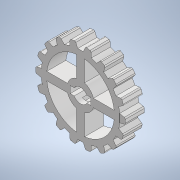
# Autodesk Inventor part: mixer_gear
Saved by Autodesk Inventor 2022 (Build 260153000, 153)
## iProperties
Created: 2022-06-21
Part Number: mixer_gear
Material: Generic
Document SubType Name: Modeling
Designer: efred
Density: 1 g/cm^3
Appearance: Default
Author: efred
Autodesk Inventor part; units mm, degrees
ref_plane "YZ Plane" through (0, 0, 0) normal (1, 0, 0) x (0, 1, 0)
ref_plane "XZ Plane" through (0, 0, 0) normal (0, 1, 0) x (-1, 0, 0)
sketch "Sketch1" plane through (0, 0, 0) normal (0, 0, 1) x (1, 0, 0)
  circle A0 centre (0, 0) radius 0.5 projected
  line L0 (-1.1547, -2) -> (-1.7321, -1) projected
  line L1 (-1.7321, -1) -> (-3.5, -1) projected
  line L2 (-3.5, -1) -> (-3.5, 1) projected
  line L3 (-3.5, 1) -> (-1.7321, 1) projected
  line L4 (-1.7321, 1) -> (-1.1547, 2) projected
  line L5 (-1.1547, 2) -> (1.1547, 2) projected
  line L6 (1.1547, 2) -> (1.7321, 1) projected
  line L7 (1.7321, 1) -> (3.5, 1) projected
  line L8 (3.5, 1) -> (3.5, -1) projected
  line L9 (3.5, -1) -> (1.7321, -1) projected
  line L10 (1.7321, -1) -> (1.1547, -2) projected
  line L11 (1.1547, -2) -> (-1.1547, -2) projected
  circle A1 centre (0, 0) radius 5
  line L12 (-3.8, -1.3) -> (-1.9053, -1.3)
  line L13 (-1.9053, -1.3) -> (-1.3279, -2.3)
  line L14 (-1.3279, -2.3) -> (1.3279, -2.3)
  line L15 (1.3279, -2.3) -> (1.9053, -1.3)
  line L16 (1.9053, -1.3) -> (3.8, -1.3)
  line L17 (3.8, -1.3) -> (3.8, 1.3)
  line L18 (3.8, 1.3) -> (1.9053, 1.3)
  line L19 (1.9053, 1.3) -> (1.3279, 2.3)
  line L20 (1.3279, 2.3) -> (-1.3279, 2.3)
  line L21 (-1.3279, 2.3) -> (-1.9053, 1.3)
  line L22 (-1.9053, 1.3) -> (-3.8, 1.3)
  line L23 (-3.8, 1.3) -> (-3.8, -1.3)
  dimension "d0" = 10
  dimension "d1" = 0.3
  constraints: 24 end point, 1 centre point, 1 coincident, 11 other
  measures "d0" diameter of A1
  measures "d1" distance between parallel lines of L1 L12
extrude "Extrusion1" add sketch "Sketch1" along normal blind 2 and the other way blind 5 contours A1
sketch "Sketch2" plane through (0, 0, -5) normal (0, 0, -1) x (-1, 0, 0)
  circle A0 centre (0, 0) radius 5 projected
  line L0 (3.8, 1.3) -> (3.8, -1.3) projected
  line L1 (3.8, -1.3) -> (1.9053, -1.3) projected
  line L2 (1.9053, -1.3) -> (1.3279, -2.3) projected
  line L3 (1.3279, -2.3) -> (-1.3279, -2.3) projected
  line L4 (-1.3279, -2.3) -> (-1.9053, -1.3) projected
  line L5 (-1.9053, -1.3) -> (-3.8, -1.3) projected
  line L6 (-3.8, -1.3) -> (-3.8, 1.3) projected
  line L7 (-3.8, 1.3) -> (-1.9053, 1.3) projected
  line L8 (-1.9053, 1.3) -> (-1.3279, 2.3) projected
  line L9 (-1.3279, 2.3) -> (1.3279, 2.3) projected
  line L10 (1.3279, 2.3) -> (1.9053, 1.3) projected
  line L11 (1.9053, 1.3) -> (3.8, 1.3) projected
  line L12 (3.8, 1.3) -> (3.8, -1.3) projected
  line L13 (3.8, 1.3) -> (3.8, -1.3)
  line L14 (3.8, -1.3) -> (1.9053, -1.3)
  line L15 (1.9053, -1.3) -> (1.3279, -2.3) projected
  line L16 (1.9053, -1.3) -> (1.3279, -2.3)
  line L17 (-1.9053, -1.3) -> (-1.3279, -2.3) projected
  line L18 (-1.3279, -2.3) -> (1.3279, -2.3)
  line L19 (1.9053, 1.3) -> (3.8, 1.3) projected
  line L20 (3.8, 1.3) -> (1.9053, 1.3)
  line L21 (1.3279, 2.3) -> (1.9053, 1.3) projected
  line L22 (1.9053, 1.3) -> (1.3279, 2.3)
  line L23 (1.3279, 2.3) -> (-1.3279, 2.3)
  line L24 (-1.3, 1.9053) -> (-2.3, 1.3279)
  line L25 (-2.3, 1.3279) -> (-2.3, -1.3279)
  line L26 (2.3, -1.3279) -> (2.3, 1.3279)
  line L27 (1.3, 1.9053) -> (2.3, 1.3279)
  line L28 (1.3, 3.8) -> (1.3, 1.9053)
  line L29 (-1.3, 3.8) -> (-1.3, 1.9053)
  line L30 (-1.3, 3.8) -> (1.3, 3.8)
  line L31 (-1.9053, -1.3) -> (-1.3279, -2.3)
  line L32 (-1.3279, -2.3) -> (1.3279, -2.3)
  line L33 (1.3279, 2.3) -> (-1.3279, 2.3)
  line L34 (-1.9053, 1.3) -> (-1.3279, 2.3)
  line L35 (-3.8, 1.3) -> (-1.9053, 1.3)
  line L36 (-3.8, -1.3) -> (-1.9053, -1.3)
  line L37 (-3.8, -1.3) -> (-3.8, 1.3)
  line L38 (1.3, -1.9053) -> (2.3, -1.3279)
  line L39 (2.3, -1.3279) -> (2.3, 1.3279)
  line L40 (-2.3, 1.3279) -> (-2.3, -1.3279)
  line L41 (-1.3, -1.9053) -> (-2.3, -1.3279)
  line L42 (-1.3, -3.8) -> (-1.3, -1.9053)
  line L43 (1.3, -3.8) -> (1.3, -1.9053)
  line L44 (1.3, -3.8) -> (-1.3, -3.8)
  point P0 (1.3, -2.3)
  point P1 (-1.3, -2.3)
  point P2 (-1.3, 2.3)
  point P3 (1.3, 2.3)
  point P4 (-2.3, 1.3)
  point P5 (-1.6837, 1.6837)
  point P6 (-1.6837, -1.6837)
  point P7 (-2.3, -1.3)
  point P8 (1.6837, -1.6837)
  point P9 (2.3, -1.3)
  point P10 (1.6837, 1.6837)
  point P11 (2.3, 1.3)
  dimension "d8" = 360
  constraints: 56 end point, 4 collinear, 1 point on line, 65 other
ref_plane "Work Plane1" through (-8.8, -2.2, 0) normal (0, 0, 1) x (1, 0, 0)
extrude "Extrusion2" cut sketch "Sketch2" against normal up to surface (5 mm away) contours L11 L10 L27 L26 | L26 L38 L2 L1 | L9 L29 L30 L28 | L43 L44 L42 L3 | L8 L7 L25 L24 | L41 L25 L5 L4
sketch "Sketch3" plane through (0, 0, -5) normal (0, 0, -1) x (-1, 0, 0)
  line L0 (-1.6837, 1.6837) -> (-2.3, 1.3279) projected
  circle A0 centre (0, 0) radius 2.6558
  constraints: 1 coincident, 3 other
extrude "Extrusion3" cut sketch "Sketch3" against normal through all
sketch "Sketch4" plane through (0, 0, -5) normal (0, 0, -1) x (-1, 0, 0)
  circle A0 centre (0, 0) radius 5 projected
  circle A1 centre (0, 0) radius 16.5 construction
  circle A2 centre (-20.3143, -27.9603) radius 16.5 construction
  circle A3 centre (0, 0) radius 14.5
  circle A4 centre (0, 0) radius 12.5
  line L0 (-14.4222, -1.5) -> (-4.7697, -1.5)
  line L1 (-4.7697, -1.5) -> (-4.7697, 1.5)
  line L2 (-4.7697, 1.5) -> (-14.4222, 1.5)
  line L3 (-14.4222, 1.5) -> (-14.4222, -1.5)
  line L4 (-5, 0) -> (-12.5, 0) construction
  line L5 (1.5, -14.4222) -> (1.5, -4.7697)
  line L6 (-1.5, -4.7697) -> (-1.5, -14.4222)
  line L7 (14.4222, 1.5) -> (4.7697, 1.5)
  line L8 (4.7697, -1.5) -> (14.4222, -1.5)
  line L9 (-1.5, 14.4222) -> (-1.5, 4.7697)
  line L10 (1.5, 4.7697) -> (1.5, 14.4222)
  line L11 (-16.1073, -1.0885) -> (-14.4222, -1.5)
  line L12 (-16.1073, 1.0885) -> (-14.4222, 1.5)
  arc A5 (-16.4883, 0.6216) -> (-16.4883, -0.6216) centre (0, 0) ccw
  arc A6 (-16.4883, -0.6216) -> (-16.1073, -1.0885) centre (-15.9886, -0.6028) ccw
  arc A7 (-16.1073, 1.0885) -> (-16.4883, 0.6216) centre (-15.9886, 0.6028) ccw
  arc A8 (-14.7602, 1.4175) -> (-14.3828, 1.8398) centre (-14.8788, 1.9032) ccw
  arc A9 (-14.3828, -1.8398) -> (-14.7602, -1.4175) centre (-14.8788, -1.9032) ccw
  arc A10 (-14.3548, -3.7163) -> (-14.1447, -3.1904) centre (-14.6324, -3.3004) ccw
  line L13 (-15.5082, -4.4861) -> (-14.0655, -3.5231)
  arc A11 (-15.5082, -4.4861) -> (-15.7065, -5.0552) centre (-15.2306, -4.902) ccw
  arc A12 (-15.7065, -5.0552) -> (-15.2813, -6.2235) centre (0, 0) ccw
  arc A13 (-15.2813, -6.2235) -> (-14.7636, -6.5319) centre (-14.8182, -6.0349) ccw
  arc A14 (-12.8862, -6.648) -> (-13.3852, -6.3803) centre (-13.3305, -6.8773) ccw
  line L14 (-14.7636, -6.5319) -> (-13.0394, -6.3422)
  arc A15 (-12.2181, -8.4018) -> (-12.2004, -7.8358) centre (-12.6212, -8.106) ccw
  line L15 (-13.0386, -9.5197) -> (-12.0122, -8.1213)
  arc A16 (-13.0386, -9.5197) -> (-13.0303, -10.1223) centre (-12.6355, -9.8155) ccw
  arc A17 (-13.0303, -10.1223) -> (-12.2312, -11.0746) centre (0, 0) ccw
  arc A18 (-12.2312, -11.0746) -> (-11.6392, -11.1874) centre (-11.8606, -10.7391) ccw
  arc A19 (-9.8353, -10.6544) -> (-10.3958, -10.5735) centre (-10.1744, -11.0218) ccw
  line L16 (-11.6392, -11.1874) -> (-10.0839, -10.4195)
  arc A20 (-8.6076, -12.0739) -> (-8.7847, -11.536) centre (-9.0876, -11.9338) ccw
  line L17 (-8.9963, -13.405) -> (-8.5101, -11.74)
  arc A21 (-8.9963, -13.405) -> (-8.7825, -13.9685) centre (-8.5163, -13.5452) ccw
  arc A22 (-8.7825, -13.9685) -> (-7.7058, -14.5901) centre (0, 0) ccw
  arc A23 (-7.7058, -14.5901) -> (-7.111, -14.4935) centre (-7.4723, -14.148) ccw
  arc A24 (-5.5981, -13.3758) -> (-6.1525, -13.4914) centre (-5.7912, -13.837) ccw
  line L18 (-7.111, -14.4935) -> (-5.9121, -13.24)
  arc A25 (-3.959, -14.2898) -> (-4.3094, -13.8448) centre (-4.458, -14.3222) ccw
  line L19 (-3.869, -15.6735) -> (-3.9816, -13.9426)
  arc A26 (-3.869, -15.6735) -> (-3.4753, -16.1299) centre (-3.37, -15.6411) ccw
  arc A27 (-3.4753, -16.1299) -> (-2.251, -16.3457) centre (0, 0) ccw
  arc A28 (-2.251, -16.3457) -> (-1.725, -16.0516) centre (-2.1828, -15.8504) ccw
  arc A29 (-0.6857, -14.4838) -> (-1.1671, -14.7821) centre (-0.7094, -14.9832) ccw
  line L20 (-1.725, -16.0516) -> (-1.0272, -14.4636)
  arc A30 (1.1671, -14.7821) -> (0.6857, -14.4838) centre (0.7094, -14.9832) ccw
  line L21 (1.725, -16.0516) -> (1.0272, -14.4636)
  arc A31 (1.725, -16.0516) -> (2.251, -16.3457) centre (2.1828, -15.8504) ccw
  arc A32 (2.251, -16.3457) -> (3.4753, -16.1299) centre (0, 0) ccw
  arc A33 (3.4753, -16.1299) -> (3.869, -15.6735) centre (3.37, -15.6411) ccw
  arc A34 (4.3094, -13.8448) -> (3.959, -14.2898) centre (4.458, -14.3222) ccw
  line L22 (3.869, -15.6735) -> (3.9816, -13.9426)
  arc A35 (6.1525, -13.4914) -> (5.5981, -13.3758) centre (5.7912, -13.837) ccw
  line L23 (7.111, -14.4935) -> (5.9121, -13.24)
  arc A36 (7.111, -14.4935) -> (7.7058, -14.5901) centre (7.4723, -14.148) ccw
  arc A37 (7.7058, -14.5901) -> (8.7825, -13.9685) centre (0, 0) ccw
  arc A38 (8.7825, -13.9685) -> (8.9963, -13.405) centre (8.5163, -13.5452) ccw
  arc A39 (8.7847, -11.536) -> (8.6076, -12.0739) centre (9.0876, -11.9338) ccw
  line L24 (8.9963, -13.405) -> (8.5101, -11.74)
  arc A40 (10.3958, -10.5735) -> (9.8353, -10.6544) centre (10.1744, -11.0218) ccw
  line L25 (11.6392, -11.1874) -> (10.0839, -10.4195)
  arc A41 (11.6392, -11.1874) -> (12.2312, -11.0746) centre (11.8606, -10.7391) ccw
  arc A42 (12.2312, -11.0746) -> (13.0303, -10.1223) centre (0, 0) ccw
  arc A43 (13.0303, -10.1223) -> (13.0386, -9.5197) centre (12.6355, -9.8155) ccw
  arc A44 (12.2004, -7.8358) -> (12.2181, -8.4018) centre (12.6212, -8.106) ccw
  line L26 (13.0386, -9.5197) -> (12.0122, -8.1213)
  arc A45 (13.3852, -6.3803) -> (12.8862, -6.648) centre (13.3305, -6.8773) ccw
  line L27 (14.7636, -6.5319) -> (13.0394, -6.3422)
  arc A46 (14.7636, -6.5319) -> (15.2813, -6.2235) centre (14.8182, -6.0349) ccw
  arc A47 (15.2813, -6.2235) -> (15.7065, -5.0552) centre (0, 0) ccw
  arc A48 (15.7065, -5.0552) -> (15.5082, -4.4861) centre (15.2306, -4.902) ccw
  arc A49 (14.1447, -3.1904) -> (14.3548, -3.7163) centre (14.6324, -3.3004) ccw
  line L28 (15.5082, -4.4861) -> (14.0655, -3.5231)
  arc A50 (14.7602, -1.4175) -> (14.3828, -1.8398) centre (14.8788, -1.9032) ccw
  line L29 (16.1073, -1.0885) -> (14.4222, -1.5)
  arc A51 (16.1073, -1.0885) -> (16.4883, -0.6216) centre (15.9886, -0.6028) ccw
  arc A52 (16.4883, -0.6216) -> (16.4883, 0.6216) centre (0, 0) ccw
  arc A53 (16.4883, 0.6216) -> (16.1073, 1.0885) centre (15.9886, 0.6028) ccw
  arc A54 (14.3828, 1.8398) -> (14.7602, 1.4175) centre (14.8788, 1.9032) ccw
  line L30 (16.1073, 1.0885) -> (14.4222, 1.5)
  arc A55 (14.3548, 3.7163) -> (14.1447, 3.1904) centre (14.6324, 3.3004) ccw
  line L31 (15.5082, 4.4861) -> (14.0655, 3.5231)
  arc A56 (15.5082, 4.4861) -> (15.7065, 5.0552) centre (15.2306, 4.902) ccw
  arc A57 (15.7065, 5.0552) -> (15.2813, 6.2235) centre (0, 0) ccw
  arc A58 (15.2813, 6.2235) -> (14.7636, 6.5319) centre (14.8182, 6.0349) ccw
  arc A59 (12.8862, 6.648) -> (13.3852, 6.3803) centre (13.3305, 6.8773) ccw
  line L32 (14.7636, 6.5319) -> (13.0394, 6.3422)
  arc A60 (12.2181, 8.4018) -> (12.2004, 7.8358) centre (12.6212, 8.106) ccw
  line L33 (13.0386, 9.5197) -> (12.0122, 8.1213)
  arc A61 (13.0386, 9.5197) -> (13.0303, 10.1223) centre (12.6355, 9.8155) ccw
  arc A62 (13.0303, 10.1223) -> (12.2312, 11.0746) centre (0, 0) ccw
  arc A63 (12.2312, 11.0746) -> (11.6392, 11.1874) centre (11.8606, 10.7391) ccw
  arc A64 (9.8353, 10.6544) -> (10.3958, 10.5735) centre (10.1744, 11.0218) ccw
  line L34 (11.6392, 11.1874) -> (10.0839, 10.4195)
  arc A65 (8.6076, 12.0739) -> (8.7847, 11.536) centre (9.0876, 11.9338) ccw
  line L35 (8.9963, 13.405) -> (8.5101, 11.74)
  arc A66 (8.9963, 13.405) -> (8.7825, 13.9685) centre (8.5163, 13.5452) ccw
  arc A67 (8.7825, 13.9685) -> (7.7058, 14.5901) centre (0, 0) ccw
  arc A68 (7.7058, 14.5901) -> (7.111, 14.4935) centre (7.4723, 14.148) ccw
  arc A69 (5.5981, 13.3758) -> (6.1525, 13.4914) centre (5.7912, 13.837) ccw
  line L36 (7.111, 14.4935) -> (5.9121, 13.24)
  arc A70 (3.959, 14.2898) -> (4.3094, 13.8448) centre (4.458, 14.3222) ccw
  line L37 (3.869, 15.6735) -> (3.9816, 13.9426)
  arc A71 (3.869, 15.6735) -> (3.4753, 16.1299) centre (3.37, 15.6411) ccw
  arc A72 (3.4753, 16.1299) -> (2.251, 16.3457) centre (0, 0) ccw
  arc A73 (2.251, 16.3457) -> (1.725, 16.0516) centre (2.1828, 15.8504) ccw
  arc A74 (0.6857, 14.4838) -> (1.1671, 14.7821) centre (0.7094, 14.9832) ccw
  line L38 (1.725, 16.0516) -> (1.0272, 14.4636)
  arc A75 (-1.1671, 14.7821) -> (-0.6857, 14.4838) centre (-0.7094, 14.9832) ccw
  line L39 (-1.725, 16.0516) -> (-1.0272, 14.4636)
  arc A76 (-1.725, 16.0516) -> (-2.251, 16.3457) centre (-2.1828, 15.8504) ccw
  arc A77 (-2.251, 16.3457) -> (-3.4753, 16.1299) centre (0, 0) ccw
  arc A78 (-3.4753, 16.1299) -> (-3.869, 15.6735) centre (-3.37, 15.6411) ccw
  arc A79 (-4.3094, 13.8448) -> (-3.959, 14.2898) centre (-4.458, 14.3222) ccw
  line L40 (-3.869, 15.6735) -> (-3.9816, 13.9426)
  arc A80 (-6.1525, 13.4914) -> (-5.5981, 13.3758) centre (-5.7912, 13.837) ccw
  line L41 (-7.111, 14.4935) -> (-5.9121, 13.24)
  arc A81 (-7.111, 14.4935) -> (-7.7058, 14.5901) centre (-7.4723, 14.148) ccw
  arc A82 (-7.7058, 14.5901) -> (-8.7825, 13.9685) centre (0, 0) ccw
  arc A83 (-8.7825, 13.9685) -> (-8.9963, 13.405) centre (-8.5163, 13.5452) ccw
  arc A84 (-8.7847, 11.536) -> (-8.6076, 12.0739) centre (-9.0876, 11.9338) ccw
  line L42 (-8.9963, 13.405) -> (-8.5101, 11.74)
  arc A85 (-10.3958, 10.5735) -> (-9.8353, 10.6544) centre (-10.1744, 11.0218) ccw
  line L43 (-11.6392, 11.1874) -> (-10.0839, 10.4195)
  arc A86 (-11.6392, 11.1874) -> (-12.2312, 11.0746) centre (-11.8606, 10.7391) ccw
  arc A87 (-12.2312, 11.0746) -> (-13.0303, 10.1223) centre (0, 0) ccw
  arc A88 (-13.0303, 10.1223) -> (-13.0386, 9.5197) centre (-12.6355, 9.8155) ccw
  arc A89 (-12.2004, 7.8358) -> (-12.2181, 8.4018) centre (-12.6212, 8.106) ccw
  line L44 (-13.0386, 9.5197) -> (-12.0122, 8.1213)
  arc A90 (-13.3852, 6.3803) -> (-12.8862, 6.648) centre (-13.3305, 6.8773) ccw
  line L45 (-14.7636, 6.5319) -> (-13.0394, 6.3422)
  arc A91 (-14.7636, 6.5319) -> (-15.2813, 6.2235) centre (-14.8182, 6.0349) ccw
  arc A92 (-15.2813, 6.2235) -> (-15.7065, 5.0552) centre (0, 0) ccw
  arc A93 (-15.7065, 5.0552) -> (-15.5082, 4.4861) centre (-15.2306, 4.902) ccw
  arc A94 (-14.1447, 3.1904) -> (-14.3548, 3.7163) centre (-14.6324, 3.3004) ccw
  line L46 (-15.5082, 4.4861) -> (-14.0655, 3.5231)
  arc A95 (-24.387, -30.8608) -> (-20.267, -32.96) centre (-20.3143, -27.9603) ccw projected
  point P0 (-16.4697, -1)
  point P1 (-16.4697, 1)
  point P2 (-16.4697, 1)
  point P3 (-12.4097, 1.5)
  point P4 (-1.5, 12.4097)
  point P5 (-1.5, 4.7697)
  point P6 (1.5, 12.4097)
  point P7 (12.4097, 1.5)
  point P8 (4.7697, 1.5)
  point P9 (12.4097, -1.5)
  point P10 (1.5, -12.4097)
  point P11 (1.5, -4.7697)
  point P12 (-1.5, -12.4097)
  point P13 (-12.4097, -1.5)
  dimension "d17" = 2
  dimension "d14" = 33
  dimension "d15" = 33
  dimension "d16" = 2
  dimension "d18" = 3
  dimension "d21" = 360
  dimension "d23" = 2
  dimension "d24" = 3
  dimension "d25" = 0.5
  dimension "d26" = 0.5
  dimension "d29" = 360
  constraints: 187 point on circle, 94 end point, 92 centre point, 20 point on line, 5 symmetric about line, 5 tangent, 2 coincident, 2 equal radius, 2 horizontal, 2 parallel, 1 horizontal alignment, 1 perpendicular, 432 other
  measures "d14" diameter of A2
  measures "d15" diameter of A1
  measures "d18" distance between parallel lines of L0 L2
  measures "d23" distance of point (-16.47, 1) A1.start
  measures "d24" distance of L11.end L12.end
  measures "d25" radius of A6
  measures "d26" radius of A8
extrude "Extrusion4" add sketch "Sketch4" against normal up to surface (7 mm away) contours A0 L7 A4 L8 | A0 L9 A4 L10 | L7 A3 L8 A4 | A4 L10 A3 L7 | L5 A4 L6 A0 | L8 A3 L5 A4 | A4 L9 A3 L10 | L30 A53 A52 A51 L29 A3 | L5 A3 L6 A4 | A0 L0 A4 L2 | A4 L2 A3 L9 | A3 L38 A73 A72 A71 L37 | L6 A3 L0 A4 | A3 L22 A33 A32 A31 L21 | A4 L0 L3 L2 | A3 L40 A78 A77 A76 L39 | A3 L20 A28 A27 A26 L19 | A3 L11 A6 A5 A7 L12 | A3 L32 A58 A57 A56 L31 | L28 A48 A47 A46 L27 A3 | L36 A68 A67 A66 L35 A3 | A3 L24 A38 A37 A36 L23 | L46 A93 A92 A91 L45 A3 | A3 L42 A83 A82 A81 L41 | A3 L14 A13 A12 A11 L13 | L18 A23 A22 A21 L17 A3 | A3 L34 A63 A62 A61 L33 | L26 A43 A42 A41 L25 A3 | L44 A88 A87 A86 L43 A3 | A3 L16 A18 A17 A16 L15
equation "\"d15\" = d14"
body "Solid1"
